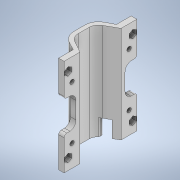
# Autodesk Inventor part: battery_2.2
Saved by Autodesk Inventor 2020 (Build 240168000, 168)
## iProperties
Created: 2022-07-16
Part Number: battery_2.2
Material: Типовые
Document SubType Name: Modeling
Designer: akapu
Density: 1 g/cm^3
Appearance: По умолчанию
Author: akapu
Autodesk Inventor part; units mm, degrees
ref_plane "YZ Plane" through (0, 0, 0) normal (1, 0, 0) x (0, 1, 0)
ref_plane "XZ Plane" through (0, 0, 0) normal (0, 1, 0) x (-1, 0, 0)
ref_plane "XY Plane" through (0, 0, 0) normal (0, 0, 1) x (1, 0, 0)
sketch "Эскиз1" plane through (0, 0, 0) normal (0, 1, 0) x (-1, 0, 0)
  line L0 (0, 0) -> (0, -8.65)
  line L1 (0, 0) -> (0, -53.5)
  line L2 (0, -53.5) -> (0, -44.85)
  line L3 (0, 0) -> (4, 0)
  line L4 (0, -53.5) -> (4.1927, -53.5)
  line L5 (0, -26.75) -> (0, -40.85)
  line L6 (0, -40.85) -> (0, -12.65)
  line L7 (0, -12.65) -> (0, -11.65)
  line L8 (0, -40.85) -> (0, -41.85)
  circle A0 centre (5.4, -22.75) radius 7
  circle A1 centre (5.4, -30.75) radius 7
  line L9 (12.4, -22.75) -> (12.4, -30.75)
  line L10 (0, -41.85) -> (8.8481, -36.8419)
  line L11 (0, -11.65) -> (8.8481, -16.6581)
  circle A2 centre (5.4, -22.75) radius 10
  circle A3 centre (5.4, -30.75) radius 10
  line L12 (15.4, -22.75) -> (15.4, -30.75)
  line L13 (0, -11.65) -> (0, -10.7122)
  line L14 (0, -11.65) -> (0, -8.65)
  line L15 (0, -41.85) -> (0, -44.85)
  line L16 (0, -8.65) -> (10.3258, -14.0473)
  line L17 (0, -44.85) -> (10.028, -39.6146)
  line L18 (4, 0) -> (4, -10.7408)
  line L19 (4.1927, -53.5) -> (4.1927, -42.6611)
  dimension "d0" = 8.65
  dimension "d1" = 53.5
  dimension "d3" = 4
  dimension "d18" = 14
  dimension "d20" = 20
  dimension "d21" = 20
  dimension "d22" = 3
  dimension "d23" = 3
  constraints: 38 end point, 8 point on circle, 7 vertical, 5 tangent, 4 centre point, 3 point on line, 2 coincident, 2 horizontal, 10 other
  measures "d0" distance of L0.start L0.end
  measures "d1" distance of L0.start L2.start
  measures "d3" distance of L0.start L3.end
  measures "d18" diameter of A0
  measures "d20" diameter of A2
  measures "d21" diameter of A3
  measures "d22" distance of L7.end L0.end
  measures "d23" distance of L8.end L2.end
extrude "Выдавливание1" add sketch "Эскиз1" along normal blind 71 contours L3 L18 L16 L0 | L16 A2 L11 L1 | L16 A2 A3 L9 A0 L11 | L12 A3 A2 | A3 L10 A1 L9 A2 | A2 L9 A3 | L17 L1 L10 A3 | L19 L4 L1 L17
sketch "Эскиз2" plane through (-4.1927, 0, -53.5) normal (-1, 0, 0) x (0, 0, 1)
  line L0 (0, 0) -> (0, 71) projected
  line L1 (0, 35.5) -> (0, 41.7)
  line L2 (0, 41.7) -> (0, 29.3)
  line L3 (53.5, 0) -> (53.5, 71) projected
  line L4 (0, 29.3) -> (53.5, 29.3)
  line L5 (53.5, 29.3) -> (53.5, 41.7)
  line L6 (53.5, 41.7) -> (0, 41.7)
  line L7 (0, 41.7) -> (0, 29.3)
  line L8 (0, 29.3) -> (8.75, 29.3)
  line L9 (8.75, 29.3) -> (8.75, 41.7)
  line L10 (53.5, 29.3) -> (44.75, 29.3)
  line L11 (44.75, 29.3) -> (44.75, 41.7)
  line L12 (0, 41.7) -> (0, 46.7)
  line L13 (0, 29.3) -> (0, 24.3)
  line L14 (0, 24.3) -> (53.5, 24.3)
  line L15 (53.5, 24.3) -> (53.5, 46.7)
  line L16 (53.5, 46.7) -> (0, 46.7)
  line L17 (0, 46.7) -> (0, 24.3)
  arc A0 (4.375, 24.3) -> (8.75, 29.3) centre (3.7502, 29.2608) ccw
  arc A1 (8.75, 41.7) -> (4.375, 46.7) centre (3.7502, 41.7392) ccw
  arc A2 (44.75, 29.3) -> (49.125, 24.3) centre (49.7498, 29.2608) ccw
  arc A3 (49.125, 46.7) -> (44.75, 41.7) centre (49.7498, 41.7392) ccw
  dimension "d26" = 6.2
  dimension "d27" = 12.4
  dimension "d28" = 8.75
  dimension "d29" = 8.75
  dimension "d30" = 5
  dimension "d31" = 5
  dimension "d33" = 5
  dimension "d34" = 5
  dimension "d35" = 5
  dimension "d36" = 5
  constraints: 32 end point, 14 point on line, 8 point on circle, 4 centre point, 4 parallel, 4 perpendicular, 2 horizontal, 1 midpoint
  measures "d26" distance of L1.start L1.end
  measures "d27" distance of L1.end L2.end
  measures "d28" distance of L2.end L8.end
  measures "d29" distance of L4.end L10.end
  measures "d30" distance of L6.end L12.end
  measures "d31" distance of L2.end L13.end
  measures "d33" radius of A0
  measures "d34" radius of A1
  measures "d35" radius of A2
  measures "d36" radius of A3
extrude "Выдавливание2" cut sketch "Эскиз2" against normal blind 10 contours L0 L4 A0 L14 | L0 L6 L9 L4 | A2 L4 L3 L14 | L0 L16 A1 L6 | L11 L6 L3 L4 | A3 L16 L3 L6
fillet "Сопряжение1" radius 2 4 edges at (-2.0964, 46.7, -53.5) (-2.0964, 24.3, -53.5) (-2, 24.3, 0) (-2, 46.7, 0)
sketch "Эскиз3" plane through (-4.1927, 0, -53.5) normal (-1, 0, 0) x (0, 0, 1)
  line L0 (0, 71) -> (10.8389, 71) projected
  line L1 (0, 71) -> (3, 71)
  line L2 (3, 71) -> (3, 63)
  line L3 (3, 63) -> (0, 63)
  line L4 (0, 63) -> (0, 71)
  line L5 (53.5, 0) -> (53.5, 22.3) projected
  line L6 (53.5, 0) -> (50.5, 0)
  line L7 (50.5, 0) -> (50.5, 8)
  line L8 (50.5, 8) -> (53.5, 8)
  line L9 (53.5, 8) -> (53.5, 0)
  line L10 (50.5, 8) -> (3, 8)
  line L11 (3, 8) -> (3, 63)
  line L12 (3, 63) -> (50.5, 63)
  line L13 (50.5, 63) -> (50.5, 8)
  line L14 (3, 63) -> (5.8, 63)
  line L15 (5.8, 63) -> (5.8, 55)
  line L16 (5.8, 55) -> (3, 55)
  line L17 (3, 55) -> (3, 63)
  line L18 (50.5, 8) -> (47.7, 8)
  line L19 (47.7, 8) -> (47.7, 16)
  line L20 (47.7, 16) -> (50.5, 16)
  line L21 (50.5, 16) -> (50.5, 8)
  line L22 (5.8, 55) -> (47.7, 55)
  line L23 (47.7, 55) -> (47.7, 16)
  line L24 (47.7, 16) -> (5.8, 16)
  line L25 (5.8, 16) -> (5.8, 55)
  line L26 (5.8, 55) -> (8.4, 55)
  line L27 (47.7, 16) -> (45.1, 16)
  line L28 (8.4, 55) -> (45.1, 55)
  line L29 (45.1, 55) -> (45.1, 16)
  line L30 (45.1, 16) -> (8.4, 16)
  line L31 (8.4, 16) -> (8.4, 55)
  line L32 (8.4, 53.4989) -> (5.8, 51.9978)
  line L33 (5.8, 51.9978) -> (3.2, 53.4989)
  line L34 (3.2, 53.4989) -> (3.2, 56.5011)
  line L35 (3.2, 56.5011) -> (5.8, 58.0022)
  line L36 (5.8, 58.0022) -> (8.4, 56.5011)
  line L37 (8.4, 56.5011) -> (8.4, 53.4989)
  line L38 (45.1, 17.5011) -> (47.7, 19.0022)
  line L39 (47.7, 19.0022) -> (50.3, 17.5011)
  line L40 (50.3, 17.5011) -> (50.3, 14.4989)
  line L41 (50.3, 14.4989) -> (47.7, 12.9978)
  line L42 (47.7, 12.9978) -> (45.1, 14.4989)
  line L43 (45.1, 14.4989) -> (45.1, 17.5011)
  line L44 (45.1, 56.5011) -> (47.7, 58.0022)
  line L45 (47.7, 58.0022) -> (50.3, 56.5011)
  line L46 (50.3, 56.5011) -> (50.3, 53.4989)
  line L47 (50.3, 53.4989) -> (47.7, 51.9978)
  line L48 (47.7, 51.9978) -> (45.1, 53.4989)
  line L49 (45.1, 53.4989) -> (45.1, 56.5011)
  line L50 (8.4, 14.4989) -> (5.8, 12.9978)
  line L51 (5.8, 12.9978) -> (3.2, 14.4989)
  line L52 (3.2, 14.4989) -> (3.2, 17.5011)
  line L53 (3.2, 17.5011) -> (5.8, 19.0022)
  line L54 (5.8, 19.0022) -> (8.4, 17.5011)
  line L55 (8.4, 17.5011) -> (8.4, 14.4989)
  point P0 (42.7592, 55)
  point P1 (6.3584, 16)
  point P2 (8.4, 53.4989)
  point P3 (8.4, 17.5011)
  dimension "d40" = 3
  dimension "d41" = 8
  dimension "d42" = 3
  dimension "d43" = 8
  dimension "d44" = 2.8
  dimension "d45" = 8
  dimension "d46" = 2.8
  dimension "d47" = 8
  dimension "d48" = 2.6
  dimension "d49" = 2.6
  dimension "d61" = 41.9
  dimension "d62" = 39
  constraints: 108 end point, 14 parallel, 7 horizontal, 7 perpendicular, 5 coincident, 4 midpoint, 3 point on line, 52 other
  measures "d40" distance of L2.end L3.end
  measures "d41" distance of L1.end L2.end
  measures "d42" distance of L7.end L8.end
  measures "d43" distance of L6.end L7.end
  measures "d44" distance of L15.end L16.end
  measures "d45" distance of L14.end L15.end
  measures "d46" distance of L19.end L20.end
  measures "d47" distance of L18.end L19.end
  measures "d48" distance of L15.end L26.end
  measures "d49" distance of L19.end L27.end
  measures "d61" distance of L15.end L22.end
  measures "d62" distance of L22.end L19.end
extrude "Выдавливание3" cut sketch "Эскиз3" against normal blind 2 contours L34 L35 L15 L16 | L16 L25 L33 L34 | L36 L37 L22 L15 | L22 L31 L32 L25 | L42 L43 L24 L19 | L19 L20 L40 L41 | L20 L23 L39 L40 | L24 L29 L38 L23 | L49 L44 L45 L46 L47 L23 L22 | L22 L23 L48 L29 | L54 L31 L24 L25 | L25 L24 L55 L50 L51 L52 L53
sketch "Эскиз4" plane through (-2.1927, 0, -53.5) normal (-1, 0, 0) x (0, 0, 1)
  line L0 (5.8, 55) -> (47.7, 55)
  line L1 (47.7, 55) -> (47.7, 16)
  line L2 (47.7, 16) -> (5.8, 16)
  line L3 (5.8, 16) -> (5.8, 55)
  circle A0 centre (5.8, 55) radius 1.6
  circle A1 centre (47.7, 55) radius 1.6
  circle A2 centre (47.7, 16) radius 1.6
  circle A3 centre (5.8, 16) radius 1.6
  dimension "d55" = 3.2
  dimension "d56" = 3.2
  dimension "d57" = 3.2
  dimension "d58" = 3.2
  constraints: 8 end point, 4 centre point, 3 coincident, 2 parallel, 1 horizontal, 1 perpendicular, 1 point on line
  measures "d55" diameter of A0
  measures "d56" diameter of A1
  measures "d57" diameter of A2
  measures "d58" diameter of A3
extrude "Выдавливание4" cut sketch "Эскиз4" against normal blind 3 contours L3 A0 L0 | L0 A0 L3 | A1 L1 L0 | L0 L1 A1 | A3 L2 L3 | L3 L2 A3 | A2 L2 L1 | L1 L2 A2
sketch "Эскиз5" plane through (0, 0, -53.5) normal (0, 0, -1) x (-1, 0, 0)
  line L0 (10.028, 0) -> (10.028, 71) projected
  line L1 (0, 0) -> (4.1927, 0) projected
  line L2 (4.1927, 0) -> (10.028, 0)
  line L3 (10.028, 0) -> (10.028, 12)
  line L4 (10.028, 12) -> (4.1927, 12)
  line L5 (4.1927, 12) -> (4.1927, 0)
  dimension "d68" = 12
  constraints: 8 end point, 2 parallel, 1 horizontal, 1 perpendicular, 1 point on line
  measures "d68" distance of L3.end L2.end
extrude "Выдавливание5" cut sketch "Эскиз5" against normal blind 30
fillet "Сопряжение2" radius 1 1 edges at (-10.028, 6, -39.6146)
fillet "Сопряжение3" radius 2 1 edges at (-10.028, 6, -36.0018)
sketch "Эскиз6" plane through (0, 0, -41.85) normal (1, 0, 0) x (0, 0, -1)
  line L0 (11.65, 0) -> (11.65, 22.3) projected
  line L1 (11.65, 0) -> (8.65, 0)
  line L2 (8.65, 0) -> (8.65, 8)
  line L3 (8.65, 8) -> (11.65, 8)
  line L4 (11.65, 8) -> (11.65, 0)
  line L5 (-41.85, 71.0642) -> (-38.85, 71.0642)
  line L6 (-38.85, 71.0642) -> (-38.85, 63.0642)
  line L7 (-38.85, 63.0642) -> (-41.85, 63.0642)
  line L8 (-41.85, 63.0642) -> (-41.85, 71.0642)
  line L9 (8.65, 8) -> (-38.85, 8)
  line L10 (-38.85, 8) -> (-38.85, 63.0642)
  line L11 (-38.85, 63.0642) -> (8.65, 63.0642)
  line L12 (8.65, 63.0642) -> (8.65, 8)
  circle A0 centre (8.65, 8) radius 1.6
  circle A1 centre (-38.85, 8) radius 1.6
  circle A2 centre (-38.85, 63.0642) radius 1.6
  circle A3 centre (8.65, 63.0642) radius 1.6
  point P0 (-41.85, 0)
  dimension "d71" = 3
  dimension "d72" = 8
  dimension "d73" = 3
  dimension "d74" = 8
  dimension "d75" = 3.2
  dimension "d76" = 3.2
  dimension "d77" = 3.2
  dimension "d78" = 3.2
  constraints: 24 end point, 6 parallel, 4 centre point, 4 coincident, 3 horizontal, 3 perpendicular
  measures "d71" distance of L2.end L3.end
  measures "d72" distance of L1.end L2.end
  measures "d73" distance of L6.end L7.end
  measures "d74" distance of L5.end L6.end
  measures "d75" diameter of A0
  measures "d76" diameter of A1
  measures "d77" diameter of A2
  measures "d78" diameter of A3
extrude "Выдавливание6" cut sketch "Эскиз6" against normal blind 30 contours A0 L2 L3 | L3 L12 A0 | A0 L9 L2 | L9 A0 L12 | A3 L11 L12 | L12 L11 A3 | A1 L10 L9 | L9 L10 A1 | A2 L10 L11 | L11 L6 A2 | A2 L7 L10 | L7 A2 L6
sketch "Эскиз7" plane through (0, 0, -41.85) normal (1, 0, 0) x (0, 0, -1)
  circle A0 centre (8.65, 8) radius 1.6 projected
  circle A1 centre (-38.85, 63.0642) radius 1.6 projected
  line L0 (8.65, 8) -> (-38.85, 8)
  line L1 (-38.85, 8) -> (-38.85, 63.0642)
  line L2 (-38.85, 63.0642) -> (8.65, 63.0642)
  line L3 (8.65, 63.0642) -> (8.65, 8)
  line L4 (8.65, 8) -> (6.05, 8)
  line L5 (-38.85, 63.0642) -> (-36.25, 63.0642)
  line L6 (6.05, 8) -> (-36.25, 8)
  line L7 (-36.25, 8) -> (-36.25, 63.0642)
  line L8 (-36.25, 63.0642) -> (6.05, 63.0642)
  line L9 (6.05, 63.0642) -> (6.05, 8)
  line L10 (6.05, 9.5011) -> (8.65, 11.0022)
  line L11 (8.65, 11.0022) -> (11.25, 9.5011)
  line L12 (11.25, 9.5011) -> (11.25, 6.4989)
  line L13 (11.25, 6.4989) -> (8.65, 4.9978)
  line L14 (8.65, 4.9978) -> (6.05, 6.4989)
  line L15 (6.05, 6.4989) -> (6.05, 9.5011)
  line L16 (-36.25, 6.4989) -> (-38.85, 4.9978)
  line L17 (-38.85, 4.9978) -> (-41.45, 6.4989)
  line L18 (-41.45, 6.4989) -> (-41.45, 9.5011)
  line L19 (-41.45, 9.5011) -> (-38.85, 11.0022)
  line L20 (-38.85, 11.0022) -> (-36.25, 9.5011)
  line L21 (-36.25, 9.5011) -> (-36.25, 6.4989)
  line L22 (-36.25, 61.5631) -> (-38.85, 60.062)
  line L23 (-38.85, 60.062) -> (-41.45, 61.5631)
  line L24 (-41.45, 61.5631) -> (-41.45, 64.5653)
  line L25 (-41.45, 64.5653) -> (-38.85, 66.0664)
  line L26 (-38.85, 66.0664) -> (-36.25, 64.5653)
  line L27 (-36.25, 64.5653) -> (-36.25, 61.5631)
  circle A2 centre (8.65, 63.0642) radius 1.6 projected
  line L28 (6.05, 64.5653) -> (8.65, 66.0664)
  line L29 (8.65, 66.0664) -> (11.25, 64.5653)
  line L30 (11.25, 64.5653) -> (11.25, 61.5631)
  line L31 (11.25, 61.5631) -> (8.65, 60.062)
  line L32 (8.65, 60.062) -> (6.05, 61.5631)
  line L33 (6.05, 61.5631) -> (6.05, 64.5653)
  point P0 (-41.85, 0)
  point P1 (6.05, 61.5631)
  point P2 (6.05, 9.5011)
  dimension "d81" = 2.6
  dimension "d82" = 2.6
  constraints: 68 end point, 4 coincident, 4 midpoint, 4 parallel, 2 horizontal, 2 perpendicular, 2 point on line, 52 other
  measures "d81" distance of L0.start L4.end
  measures "d82" distance of L1.end L5.end
extrude "Выдавливание7" cut sketch "Эскиз7" against normal blind 3 contours A0 L0 L3 | A0 L3 L11 L12 L13 L14 L15 L0 | L3 L0 A0 | A0 L0 L9 L10 L3 | L32 L9 L2 A2 L3 | L3 A2 L2 L33 L28 L29 L30 L31 | L21 L16 L17 L18 L19 L1 L0 | L0 L1 L20 L7 | A2 L2 L3 | L3 L2 A2 | L22 L1 A1 L2 L7 | L2 A1 L1 L23 L24 L25 L26 L27 | L2 L1 A1 | A1 L1 L2
